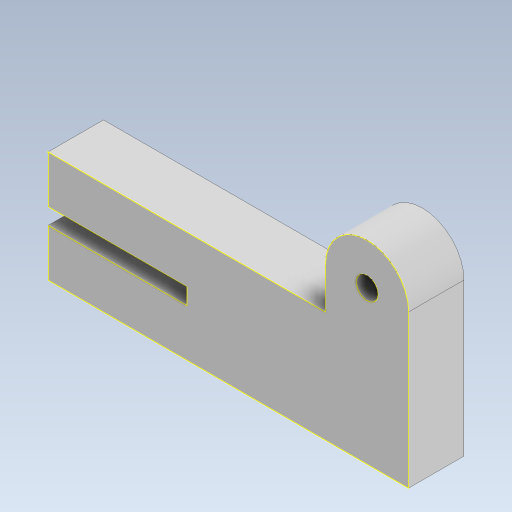
# Autodesk Inventor part: 零件7
Saved by Autodesk Inventor 2023 (Build 270158000, 158)
## iProperties
Created: 2023-05-12
Part Number: 零件7
Material: 一般
Document SubType Name: Modeling
Designer: Johnny Jou
Density: 1 g/cm^3
Appearance: 預設
Author: Johnny Jou
Autodesk Inventor part; units mm, degrees
ref_plane "YZ Plane" through (0, 0, 0) normal (1, 0, 0) x (0, 1, 0)
ref_plane "XZ Plane" through (0, 0, 0) normal (0, 1, 0) x (-1, 0, 0)
ref_plane "XY Plane" through (0, 0, 0) normal (0, 0, 1) x (1, 0, 0)
sketch "草圖1" plane through (0, 0, 0) normal (0, 0, 1) x (1, 0, 0)
  line L0 (0, 0) -> (50, 0)
  line L1 (50, -20) -> (0, -20)
  line L2 (0, -20) -> (0, 0)
  line L3 (0, -8.525) -> (25, -8.525)
  line L4 (25, -8.525) -> (25, -11.475)
  line L5 (25, -11.475) -> (0, -11.475)
  line L6 (0, -11.475) -> (0, -8.525)
  line L7 (50, 0) -> (60, 0)
  line L8 (50, 0) -> (50, -20)
  line L9 (50, -20) -> (65, -20)
  line L10 (65, -20) -> (65, 15)
  line L11 (65, 15) -> (50, 15)
  line L12 (50, 15) -> (50, -20)
  circle A0 centre (57.5, 7.5) radius 7.5
  circle A1 centre (57.5, 7.5) radius 1.975
  point P0 (25, -10)
  point P1 (0, -10)
  point P2 (65, 7.5)
  point P3 (50, 7.5)
  dimension "d0" = 20
  dimension "d2" = 25
  dimension "d3" = 2.95
  dimension "d4" = 0
  dimension "d7" = 50
  dimension "d8" = 15
  dimension "d9" = 3.95
  constraints: 26 end point, 5 parallel, 4 horizontal, 4 tangent, 3 perpendicular, 2 centre point, 2 midpoint, 1 coincident, 1 point on line
  measures "d0" distance between parallel lines of L1 L0
  measures "d2" distance of L3.start L3.end
  measures "d3" distance of L3.end L4.end
  measures "d4" vertical distance of point (25, -10) point (0, -10)
  measures "d7" distance between parallel lines of L2 L8
  measures "d8" diameter of A0
  measures "d9" diameter of A1
extrude "擠出1" add sketch "草圖1" along normal blind 10 contours L0 L8 L1 L2 L5 L4 L3 | L12 A0 L7 | L7 A0 L10 L9 L8 | A0
sketch "草圖2" plane through (0, 0, 10) normal (0, 0, 1) x (1, 0, 0)
  line L0 (0, -20) -> (65, -20) projected
  line L1 (65, -20) -> (65, 7.5) projected
  arc A0 (65, 7.5) -> (50, 7.5) centre (57.5, 7.5) ccw projected
  line L2 (50, 7.5) -> (50, 0) projected
  line L3 (50, 0) -> (0, 0) projected
  line L4 (0, 0) -> (0, -8.525) projected
  line L5 (0, -8.525) -> (25, -8.525) projected
  line L6 (25, -8.525) -> (25, -11.475) projected
  line L7 (25, -11.475) -> (0, -11.475) projected
  line L8 (0, -11.475) -> (0, -20) projected
  circle A1 centre (57.5, 7.5) radius 1.975 projected
